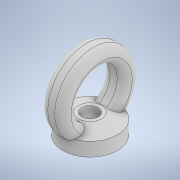
# Autodesk Inventor part: Wire holder
Saved by Autodesk Inventor 2020.2 (Build 242310000, 310)
## iProperties
Created: 2020-01-20
Part Number: Wire holder
Material: Generic
Document SubType Name: Modeling
Designer: Paul Lefeuvre
Density: 1 g/cm^3
Appearance: Default
Author: Paul Lefeuvre
Autodesk Inventor part; units mm, degrees
ref_plane "YZ Plane" through (0, 0, 0) normal (1, 0, 0) x (0, 1, 0)
ref_plane "XZ Plane" through (0, 0, 0) normal (0, 1, 0) x (-1, 0, 0)
ref_plane "XY Plane" through (0, 0, 0) normal (0, 0, 1) x (1, 0, 0)
sketch "Sketch1" plane through (0, 0, 0) normal (1, 0, 0) x (0, 1, 0)
  circle A0 centre (0, 0) radius 8.6
  circle A1 centre (0, 0) radius 14.1
  line L0 (0, 0) -> (-23.4423, 0)
  line L1 (-9.1, 10) -> (-14.1, 10)
  line L2 (-14.1, 10) -> (-14.1, -10)
  line L3 (-14.1, -10) -> (-9.1, -10)
  line L4 (-9.1, 10) -> (-6.9895, 4.2014)
  line L5 (-6.9895, 4.2014) -> (-6.9895, -4.2014)
  line L6 (-6.9895, -4.2014) -> (-9.1, -10)
  line L7 (-6.9895, 3) -> (-14.1, 3)
  line L8 (-14.1, -3) -> (-6.9895, -3)
  point P0 (-6.9895, 0)
  point P1 (-14.1, 0)
  dimension "d0" = 17.2
  dimension "d1" = 5.5
  dimension "d10" = 90
  dimension "d11" = 10
  dimension "d12" = 10
  dimension "d13" = 90
  dimension "d14" = 110
  dimension "d15" = 110
  dimension "d16" = 5
  dimension "d22" = 6
  constraints: 18 end point, 4 point on line, 2 centre point, 2 equal length, 2 perpendicular, 1 coincident, 1 horizontal, 1 tangent, 1 vertical, 1 other
  measures "d0" diameter of A0
  measures "d1" radial gap between concentric circles of A0 A1
  measures "d10" angle of L1 L2
  measures "d11" distance from line of L1.end L0
  measures "d12" distance from line of L0 L2.end
  measures "d13" angle of L2 L3
  measures "d14" angle of L1 L4
  measures "d15" angle of L3 L6
  measures "d16" distance of L2.end L3.end
  measures "d22" distance between parallel lines of L7 L8
extrude "Extrusion1" add sketch "Sketch1" along normal mid plane 8.5 contours A0 L4 L1 A1 L3 L6 | A0 L7 A1 L1 L4 | L6 L3 A1 L8 A0 | A0 L0 A1 L7 | L8 A1 L0 A0
fillet "Fillet1" radius 3 4 edges at (4.25, -14.1, 0) (-4.25, -14.1, 0) (4.25, -8.6, 0) (-4.25, -8.6, 0)
revolve "Revolution1" add sketch "Sketch1" angle 360 about axis through (0, 0, 0) along (0, -1, 0) contours L6 L3 A1 L8 A0 | A0 L8 L5 L6 | A1 L3 L2 L8
revolve "Revolution2" cut sketch "Sketch1" angle 360 about axis through (0, 0, 0) along (0, -1, 0) contours L8 A1 L0 A0 | A0 L0 L5 L8 | L8 L2 A1
equation "\"d12\" = d11"
equation "\"d15\" = d14"
body "Solid1"
